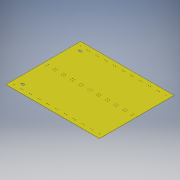
# Autodesk Inventor part: PRT1001-214 Base
Saved by Autodesk Inventor 2019 (Build 230136000, 136)
## iProperties
Created: 2019-07-02
Part Number: PRT1001-214 Base
Material: Generic
Document SubType Name: Modeling
Designer: james
Density: 1 g/cm^3
Appearance: Rubber - Black(1)
Author: james
Autodesk Inventor part; units mm, degrees
ref_plane "YZ Plane" through (0, 0, 0) normal (1, 0, 0) x (0, 1, 0)
ref_plane "XZ Plane" through (0, 0, 0) normal (0, 1, 0) x (-1, 0, 0)
ref_plane "XY Plane" through (0, 0, 0) normal (0, 0, 1) x (1, 0, 0)
sketch "Sketch3" plane through (0, 0, 0) normal (0, 1, 0) x (-1, 0, 0)
  line L0 (447.8905, 95.355) -> (-108.1095, 95.355)
  line L1 (-108.1095, 95.355) -> (-108.1095, -348.645)
  line L2 (-108.1095, -348.645) -> (447.8905, -348.645)
  line L3 (447.8905, -348.645) -> (447.8905, 95.355)
  point P0 (0, 0)
  dimension "d19" = 444
  dimension "d441" = 556
  constraints: 8 end point, 2 parallel, 1 horizontal, 1 perpendicular
  measures "d19" distance of L0.end L1.end
  measures "d441" distance between parallel lines of L3 L1
extrude "Extrusion2" add sketch "Sketch3" along normal blind 1
sketch "Sketch9" plane through (0, 1, 0) normal (0, 1, 0) x (1, 0, 0)
  line L0 (108.1095, 348.645) -> (-447.8905, 348.645) projected
  line L1 (108.1095, -95.355) -> (108.1095, 348.645) projected
  line L2 (-447.8905, -95.355) -> (108.1095, -95.355) projected
  point P0 (0, 0)
  point P1 (84.1095, 324.645)
  point P2 (44.1095, 324.645)
  point P3 (84.1095, 132.645)
  point P4 (44.1095, 132.645)
  point P5 (84.1095, 120.645)
  point P6 (84.1095, -71.355)
  point P7 (32.1095, 324.645)
  point P8 (32.1095, 132.645)
  point P9 (44.1095, 120.645)
  point P10 (32.1095, 120.645)
  point P11 (44.1095, -71.355)
  point P12 (32.1095, -71.355)
  point P13 (-7.8905, 324.645)
  point P14 (-19.8905, 324.645)
  point P15 (-59.8905, 324.645)
  point P16 (-71.8905, 324.645)
  point P17 (-111.8905, 324.645)
  point P18 (-7.8905, 132.645)
  point P19 (-7.8905, 120.645)
  point P20 (-7.8905, -71.355)
  point P21 (-19.8905, 132.645)
  point P22 (-59.8905, 132.645)
  point P23 (-123.8905, 324.645)
  point P24 (-163.8905, 324.645)
  point P25 (-175.8905, 324.645)
  point P26 (-215.8905, 324.645)
  point P27 (-215.8905, 324.645)
  point P28 (-227.8905, 324.645)
  point P29 (-267.8905, 324.645)
  point P30 (-279.8905, 324.645)
  point P31 (-319.8905, 324.645)
  point P32 (-331.8905, 324.645)
  point P33 (-371.8905, 324.645)
  point P34 (-383.8905, 324.645)
  point P35 (-423.8905, 324.645)
  point P36 (-59.8905, 132.645)
  point P37 (-71.8905, 132.645)
  point P38 (-111.8905, 132.645)
  point P39 (-123.8905, 132.645)
  point P40 (-163.8905, 132.645)
  point P41 (-267.8905, 132.645)
  point P42 (-227.8905, 132.645)
  point P43 (-215.8905, 132.645)
  point P44 (-175.8905, 132.645)
  point P45 (-163.8905, 132.645)
  point P46 (-279.8905, 132.645)
  point P47 (-319.8905, 132.645)
  point P48 (-331.8905, 132.645)
  point P49 (-371.8905, 132.645)
  point P50 (-59.8905, 120.645)
  point P51 (-71.8905, 120.645)
  point P52 (-111.8905, 120.645)
  point P53 (-123.8905, 120.645)
  point P54 (-163.8905, 120.645)
  point P55 (-267.8905, 120.645)
  point P56 (-227.8905, 120.645)
  point P57 (-215.8905, 120.645)
  point P58 (-175.8905, 120.645)
  point P59 (-163.8905, 120.645)
  point P60 (-279.8905, 120.645)
  point P61 (-319.8905, 120.645)
  point P62 (-331.8905, 120.645)
  point P63 (-371.8905, 120.645)
  point P64 (-59.8905, -71.355)
  point P65 (-71.8905, -71.355)
  point P66 (-111.8905, -71.355)
  point P67 (-123.8905, -71.355)
  point P68 (-163.8905, -71.355)
  point P69 (-267.8905, -71.355)
  point P70 (-227.8905, -71.355)
  point P71 (-215.8905, -71.355)
  point P72 (-175.8905, -71.355)
  point P73 (-163.8905, -71.355)
  point P74 (-279.8905, -71.355)
  point P75 (-319.8905, -71.355)
  point P76 (-331.8905, -71.355)
  point P77 (-371.8905, -71.355)
  point P78 (-19.8905, -71.355)
  point P79 (-19.8905, 120.645)
  point P80 (-383.8905, 132.645)
  point P81 (-423.8905, 132.645)
  point P82 (-423.8905, 120.645)
  point P83 (-383.8905, 120.645)
  point P84 (-383.8905, -71.355)
  point P85 (-423.8905, -71.355)
  dimension "d442" = 24
  dimension "d443" = 24
  dimension "d444" = 0
  dimension "d445" = 40
  dimension "d446" = 0
  dimension "d447" = 192
  dimension "d448" = 0
  dimension "d449" = 0
  dimension "d450" = 12
  dimension "d451" = 0
  dimension "d452" = 0
  dimension "d453" = 192
  dimension "d454" = 24
  dimension "d455" = 12
  dimension "d456" = 0
  dimension "d457" = 0
  dimension "d458" = 0
  dimension "d459" = 0
  dimension "d460" = 0
  dimension "d461" = 0
  dimension "d462" = 0
  dimension "d463" = 0
  dimension "d464" = 0
  dimension "d465" = 0
  dimension "d466" = 0
  dimension "d467" = 0
  dimension "d468" = 40
  dimension "d469" = 0
  dimension "d470" = 12
  dimension "d471" = 0
  dimension "d472" = 40
  dimension "d473" = 0
  dimension "d474" = 12
  dimension "d475" = 0
  dimension "d476" = 40
  dimension "d477" = 0
  dimension "d478" = 0
  dimension "d479" = 0
  dimension "d480" = 0
  dimension "d481" = 0
  dimension "d482" = 0
  dimension "d484" = 0
  dimension "d485" = 0
  dimension "d486" = 0
  dimension "d487" = 0
  dimension "d488" = 0
  dimension "d489" = 12
  dimension "d490" = 0
  dimension "d491" = 40
  dimension "d492" = 0
  dimension "d493" = 12
  dimension "d494" = 0
  dimension "d495" = 40
  dimension "d496" = 0
  dimension "d497" = 12
  dimension "d498" = 0
  dimension "d499" = 40
  dimension "d500" = 0
  dimension "d501" = 12
  dimension "d502" = 0
  dimension "d503" = 40
  dimension "d507" = 0
  dimension "d508" = 0
  dimension "d509" = 0
  measures "d442" distance from line of L0 point (84.11, 324.645)
  measures "d443" distance from line of L1 point (84.11, 324.645)
  measures "d444" vertical distance of point (84.11, 324.645) point (44.11, 324.645)
  measures "d445" distance of point (84.11, 324.645) point (44.11, 324.645)
  measures "d446" horizontal distance of point (84.11, 132.645) point (84.11, 324.645)
  measures "d447" distance of point (84.11, 324.645) point (84.11, 132.645)
  measures "d448" horizontal distance of point (44.11, 132.645) point (44.11, 324.645)
  measures "d449" vertical distance of point (84.11, 132.645) point (44.11, 132.645)
  measures "d450" distance of point (84.11, 120.645) point (84.11, 132.645)
  measures "d451" horizontal distance of point (84.11, 120.645) point (84.11, 132.645)
  measures "d452" horizontal distance of point (84.11, -71.355) point (84.11, 120.645)
  measures "d453" distance of point (84.11, 120.645) point (84.11, -71.355)
  measures "d454" distance from line of L2 point (84.11, -71.355)
  measures "d455" distance of point (44.11, 324.645) point (32.11, 324.645)
  measures "d456" vertical distance of point (32.11, 324.645) point (44.11, 324.645)
  measures "d457" horizontal distance of point (32.11, 132.645) point (32.11, 324.645)
  measures "d458" vertical distance of point (44.11, 132.645) point (32.11, 132.645)
  measures "d459" vertical distance of point (44.11, 120.645) point (84.11, 120.645)
  measures "d460" horizontal distance of point (44.11, 132.645) point (44.11, 120.645)
  measures "d461" horizontal distance of point (32.11, 120.645) point (32.11, 132.645)
  measures "d462" vertical distance of point (44.11, 120.645) point (32.11, 120.645)
  measures "d463" vertical distance of point (44.11, -71.355) point (84.11, -71.355)
  measures "d464" horizontal distance of point (44.11, -71.355) point (44.11, 120.645)
  measures "d465" vertical distance of point (44.11, -71.355) point (32.11, -71.355)
  measures "d466" horizontal distance of point (32.11, 120.645) point (32.11, -71.355)
  measures "d467" vertical distance of point (32.11, 324.645) point (-7.89, 324.645)
  measures "d468" distance of point (32.11, 324.645) point (-7.89, 324.645)
  measures "d469" vertical distance of point (-19.89, 324.645) point (-7.89, 324.645)
  measures "d470" distance of point (-7.89, 324.645) point (-19.89, 324.645)
  measures "d471" vertical distance of point (-59.89, 324.645) point (-19.89, 324.645)
  measures "d472" distance of point (-19.89, 324.645) point (-59.89, 324.645)
  measures "d473" vertical distance of point (-71.89, 324.645) point (-59.89, 324.645)
  measures "d474" distance of point (-59.89, 324.645) point (-71.89, 324.645)
  measures "d475" vertical distance of point (-71.89, 324.645) point (-111.89, 324.645)
  measures "d476" distance of point (-71.89, 324.645) point (-111.89, 324.645)
  measures "d477" horizontal distance of point (-7.89, 132.645) point (-7.89, 324.645)
  measures "d478" vertical distance of point (-7.89, 132.645) point (32.11, 132.645)
  measures "d479" vertical distance of point (32.11, 120.645) point (-7.89, 120.645)
  measures "d480" horizontal distance of point (-7.89, 132.645) point (-7.89, 120.645)
  measures "d481" vertical distance of point (32.11, -71.355) point (-7.89, -71.355)
  measures "d482" horizontal distance of point (-7.89, -71.355) point (-7.89, 120.645)
  measures "d484" horizontal distance of point (-19.89, 132.645) point (-19.89, 324.645)
  measures "d485" vertical distance of point (-7.89, 132.645) point (-19.89, 132.645)
  measures "d486" horizontal distance of point (-59.89, 132.645) point (-59.89, 324.645)
  measures "d487" vertical distance of point (-19.89, 132.645) point (-59.89, 132.645)
  measures "d488" vertical distance of point (-111.89, 324.645) point (-123.89, 324.645)
  measures "d489" distance of point (-111.89, 324.645) point (-123.89, 324.645)
  measures "d490" vertical distance of point (-123.89, 324.645) point (-163.89, 324.645)
  measures "d491" distance of point (-123.89, 324.645) point (-163.89, 324.645)
  measures "d492" vertical distance of point (-163.89, 324.645) point (-175.89, 324.645)
  measures "d493" distance of point (-163.89, 324.645) point (-175.89, 324.645)
  measures "d494" vertical distance of point (-175.89, 324.645) point (-215.89, 324.645)
  measures "d495" distance of point (-175.89, 324.645) point (-215.89, 324.645)
  measures "d496" vertical distance of point (-215.89, 324.645) point (-227.89, 324.645)
  measures "d497" distance of point (-215.89, 324.645) point (-227.89, 324.645)
  measures "d498" vertical distance of point (-227.89, 324.645) point (-267.89, 324.645)
  measures "d499" distance of point (-227.89, 324.645) point (-267.89, 324.645)
  measures "d500" vertical distance of point (-267.89, 324.645) point (-279.89, 324.645)
  measures "d501" distance of point (-267.89, 324.645) point (-279.89, 324.645)
  measures "d502" vertical distance of point (-279.89, 324.645) point (-319.89, 324.645)
  measures "d503" distance of point (-279.89, 324.645) point (-319.89, 324.645)
  measures "d507" distance of point (-215.89, 324.645) point (-215.89, 324.645)
  measures "d508" distance of point (-215.89, 324.645) point (-215.89, 324.645)
  measures "d509" vertical distance of point (-319.89, 324.645) point (-331.89, 324.645)
hole "Hole5" at (84.1095, 1, -324.645) at (44.1095, 1, -324.645) at (84.1095, 1, -132.645) at (44.1095, 1, -132.645) at (84.1095, 1, -120.645) at (84.1095, 1, 71.355) at (32.1095, 1, -324.645) at (32.1095, 1, -132.645) at (44.1095, 1, -120.645) at (32.1095, 1, -120.645) at (44.1095, 1, 71.355) at (32.1095, 1, 71.355) at (-7.8905, 1, -324.645) at (-19.8905, 1, -324.645) at (-59.8905, 1, -324.645) at (-71.8905, 1, -324.645) at (-111.8905, 1, -324.645) at (-7.8905, 1, -132.645) at (-7.8905, 1, -120.645) at (-7.8905, 1, 71.355) at (-19.8905, 1, -132.645) at (-59.8905, 1, -132.645) at (-123.8905, 1, -324.645) at (-163.8905, 1, -324.645) at (-175.8905, 1, -324.645) at (-215.8905, 1, -324.645) at (-319.8905, 1, -324.645) at (-279.8905, 1, -324.645) at (-267.8905, 1, -324.645) at (-227.8905, 1, -324.645) at (-331.8905, 1, -324.645) at (-371.8905, 1, -324.645) at (-383.8905, 1, -324.645) at (-423.8905, 1, -324.645) at (-371.8905, 1, -132.645) at (-331.8905, 1, -132.645) at (-319.8905, 1, -132.645) at (-279.8905, 1, -132.645) at (-163.8905, 1, -132.645) at (-175.8905, 1, -132.645) at (-215.8905, 1, -132.645) at (-227.8905, 1, -132.645) at (-267.8905, 1, -132.645) at (-123.8905, 1, -132.645) at (-111.8905, 1, -132.645) at (-71.8905, 1, -132.645) at (-371.8905, 1, -120.645) at (-331.8905, 1, -120.645) at (-319.8905, 1, -120.645) at (-279.8905, 1, -120.645) direction (0, -1, 0) diameter 3 end through all and at (-163.8905, 1, -120.645) (-175.8905, 1, -120.645) (-215.8905, 1, -120.645) (-227.8905, 1, -120.645) (-267.8905, 1, -120.645) (-123.8905, 1, -120.645) (-111.8905, 1, -120.645) (-71.8905, 1, -120.645) (-59.8905, 1, -120.645) (-371.8905, 1, 71.355) (-331.8905, 1, 71.355) (-319.8905, 1, 71.355) (-279.8905, 1, 71.355) (-163.8905, 1, 71.355) (-175.8905, 1, 71.355) (-215.8905, 1, 71.355) (-227.8905, 1, 71.355) (-267.8905, 1, 71.355) (-123.8905, 1, 71.355) (-111.8905, 1, 71.355) (-71.8905, 1, 71.355) (-59.8905, 1, 71.355) (-19.8905, 1, 71.355) (-19.8905, 1, -120.645) (-383.8905, 1, -132.645) (-423.8905, 1, -132.645) (-423.8905, 1, -120.645) (-383.8905, 1, -120.645) (-383.8905, 1, 71.355) (-423.8905, 1, 71.355)
sketch "Sketch11" plane through (0, 1, 0) normal (0, 1, 0) x (1, 0, 0)
  arc A0 (-402.6867, -47.5557) -> (-402.6867, -41.5542) centre (-397.0905, -44.555) ccw
  arc A1 (-402.5897, 294.67) -> (-402.5897, 301.02) centre (-397.0905, 297.845) ccw
  line L0 (108.1095, 348.645) -> (-447.8905, 348.645) projected
  line L1 (-447.8905, 348.645) -> (-447.8905, -95.355) projected
  line L2 (-447.8905, -95.355) -> (108.1095, -95.355) projected
  arc A2 (-407.2505, -41.5542) -> (-407.2505, -47.5557) centre (-407.2505, -44.555) ccw
  line L3 (-407.2505, -47.5557) -> (-402.6867, -47.5557)
  line L4 (-407.2505, -41.5542) -> (-402.6867, -41.5542)
  arc A3 (-407.2505, 301.02) -> (-407.2505, 294.67) centre (-407.2505, 297.845) ccw
  line L5 (-407.2505, 294.67) -> (-402.5897, 294.67)
  line L6 (-407.2505, 301.02) -> (-402.5897, 301.02)
  point P0 (0, 0)
  dimension "d642" = 12.7
  dimension "d643" = 50.8
  dimension "d644" = 50.8
  dimension "d645" = 50.8
  dimension "d646" = 50.8
  dimension "d647" = 12.7
  dimension "d648" = 0
  dimension "d649" = 10.16
  dimension "d650" = 0
  dimension "d651" = 10.16
  dimension "d652" = 6.35
  constraints: 8 end point, 8 point on circle, 4 centre point, 4 horizontal, 3 tangent
  measures "d642" diameter of A1
  measures "d643" distance from line of A1.centre L0
  measures "d644" distance from line of L1 A1.centre
  measures "d645" distance from line of L2 A0.centre
  measures "d646" distance from line of L1 A0.centre
  measures "d647" diameter of A0
  measures "d648" vertical distance of A2.centre A0.centre
  measures "d649" distance of A0.centre A2.centre
  measures "d650" vertical distance of A1.centre A3.centre
  measures "d651" distance of A1.centre A3.centre
  measures "d652" diameter of A3
extrude "Extrusion5" cut sketch "Sketch11" against normal blind 25.4
equation "\"d21\" = BoardHeight"
equation "\"BoardLength\" = 556"
equation "\"BoardWidth\" = 48"
equation "\"ScrewSize\" = 3"
equation "\"ScrewHoleOffset\" = 4"
equation "\"BoardGap\" = 4"
equation "\"BoardHeight\" = 1"
equation "\"BaseWidth\" = 556"
equation "\"HorizOffsetBetweenScrews\" = 192"
equation "\"BaseLength\" = 648"
equation "\"d47\" = 38"
equation "\"d55\" = 38"
equation "\"d83\" = 38"
equation "\"d85\" = 38"
equation "\"d87\" = 38"
equation "\"d88\" = 4"
equation "\"d138\" = 38"
equation "\"d140\" = 38"
equation "\"d142\" = 38"
equation "\"d143\" = 4"
equation "\"d145\" = 38"
equation "\"d147\" = 38"
equation "\"d149\" = 38"
equation "\"d150\" = 4"
equation "\"d248\" = 38"
equation "\"d250\" = 38"
equation "\"d252\" = 38"
equation "\"d253\" = 4"
equation "\"d255\" = 38"
equation "\"d257\" = 38"
equation "\"d259\" = 38"
equation "\"d260\" = 4"
equation "\"d262\" = 38"
equation "\"d264\" = 38"
equation "\"d266\" = 38"
equation "\"d267\" = 4"
equation "\"d269\" = 38"
equation "\"d271\" = 38"
equation "\"d273\" = 38"
equation "\"d274\" = 4"
equation "\"d370\" = 38"
equation "\"d372\" = 38"
equation "\"d374\" = 38"
equation "\"d375\" = 4"
equation "\"d377\" = 38"
equation "\"d379\" = 38"
equation "\"d381\" = 38"
equation "\"d382\" = 4"
equation "\"d384\" = 38"
equation "\"d386\" = 38"
equation "\"d388\" = 38"
equation "\"d389\" = 4"
equation "\"d391\" = 38"
equation "\"d393\" = 38"
equation "\"d395\" = 38"
equation "\"d396\" = 4"
equation "\"TwoBoardWidth\" = 444"
equation "\"NumberOfRows\" = 254"
equation "\"NumberOfGaps\" = 228.6"
equation "\"d505\" = 4"
equation "\"d506\" = 4"
equation "\"d545\" = 4"
equation "\"d546\" = 4"
equation "\"d547\" = 4"
equation "\"d548\" = 4"
equation "\"d579\" = 4"
equation "\"d580\" = 4"
equation "\"d581\" = 4"
equation "\"d582\" = 4"
equation "\"d613\" = 4"
equation "\"d614\" = 4"
equation "\"d615\" = 4"
equation "\"d616\" = 4"
body "Solid2"
